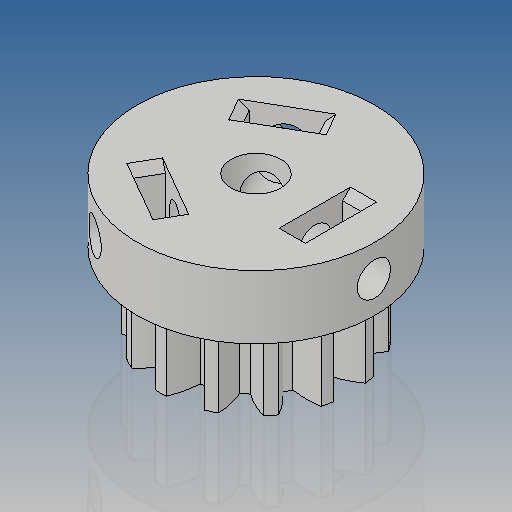
# Autodesk Inventor part: polea
Saved by Autodesk Inventor 2017 (Build 210142000, 142)
## iProperties
Part Number: polea
Material: Genérico
Document SubType Name: Modeling
Designer: Leo
Density: 1 g/cm^3
Appearance: Valor por defecto
Author: Leo
Autodesk Inventor part; units mm, degrees
ref_plane "YZ Plane" through (0, 0, 0) normal (1, 0, 0) x (0, 1, 0)
ref_plane "XZ Plane" through (0, 0, 0) normal (0, 1, 0) x (-1, 0, 0)
ref_plane "XY Plane" through (0, 0, 0) normal (0, 0, 1) x (1, 0, 0)
sketch "Boceto1" plane through (0, 0, 0) normal (0, 1, 0) x (-1, 0, 0)
  circle A0 centre (0, 0) radius 3.15
  circle A1 centre (0, 0) radius 15
  line L0 (-7.425, 3.5) -> (-10.725, 3.5)
  line L1 (-10.725, 3.5) -> (-10.725, -3.5)
  line L2 (-10.725, -3.5) -> (-7.425, -3.5)
  line L3 (-7.425, -3.5) -> (-7.425, 3.5)
  circle A2 centre (0, 0) radius 9.7265 construction
  line L4 (6.7436, -4.6802) -> (0.6814, -8.1802)
  line L5 (8.3936, -7.5381) -> (6.7436, -4.6802)
  line L6 (2.3314, -11.0381) -> (8.3936, -7.5381)
  line L7 (0.6814, -8.1802) -> (2.3314, -11.0381)
  line L8 (0.6814, 8.1802) -> (6.7436, 4.6802)
  line L9 (2.3314, 11.0381) -> (0.6814, 8.1802)
  line L10 (8.3936, 7.5381) -> (2.3314, 11.0381)
  line L11 (6.7436, 4.6802) -> (8.3936, 7.5381)
  point P0 (-7.425, 0)
  point P1 (-9.075, 3.5)
  point P2 (3.7125, -6.4302)
  point P3 (1.5064, -9.6092)
  point P4 (3.7125, 6.4302)
  point P5 (7.5686, 6.1092)
  dimension "d0" = 6.3
  dimension "tuerca" = 7
  dimension "d2" = 11.85
  dimension "d3" = 6.5765
  dimension "d4" = 3.3
  dimension "d18" = 360
  dimension "d26" = 30
  dimension "d27" = 4.275
  dimension "d28" = 4.275
  constraints: 24 end point, 2 centre point, 2 coincident, 2 midpoint, 2 parallel, 1 horizontal, 1 horizontal alignment, 1 perpendicular, 34 other
  measures "d0" diameter of A0
  measures "tuerca" distance of L0.end L1.end
  measures "d2" radial gap between concentric circles of A1 A0
  measures "d4" distance of L0.start L0.end
  measures "d26" diameter of A1
  measures "d27" distance edge to line of A0 L3
  measures "d28" distance edge to line of A1 L1
extrude "Extrusión1" add sketch "Boceto1" along normal blind 8
sketch "Boceto2" plane through (7.425, 0, -3.5) normal (1, 0, 0) x (0, 0, -1)
  line L0 (0, 0) -> (-7, 0) projected
  line L1 (0, 0) -> (0, 8) construction
  line L2 (-7, 8) -> (0, 8) construction
  line L3 (-7, 0) -> (-7, 8) construction
  line L4 (-7, 0) -> (0, 8) construction
  circle A0 centre (-3.5, 4) radius 2.1
  line L5 (0, 1.7483) -> (-3.0282, 0)
  line L6 (-3.9718, 0) -> (-7, 1.7483)
  line L7 (-7, 1.7483) -> (-7, 0)
  line L8 (0, 1.7483) -> (0, 0)
  point P0 (-3.5, 0)
  dimension "d7" = 4.2
  dimension "d8" = 120
  dimension "d9" = 3.7
  constraints: 10 end point, 4 point on line, 1 centre point, 1 collinear, 1 equal length, 1 horizontal alignment, 1 midpoint
  measures "d7" diameter of A0
  measures "d8" angle of L5 L6
  measures "d9" distance from line of A0.centre L5
extrude "Extrusión2" cut sketch "Boceto2" along normal mid plane 16 contours A0
extrude "Extrusión3" add sketch "Boceto2" along normal up to next contours L0 L5 L8 | L0 L7 L6
sketch "Boceto3" plane through (0, 0, 0) normal (0, -1, 0) x (1, 0, 0)
  circle A0 centre (0, 0) radius 3.15 projected
  circle A1 centre (0, 0) radius 17.939
  constraints: 1 centre point
extrude "Extrusión4" add sketch "Boceto3" along normal blind 10
spur gear teeth "iFeature1:3" teeth 14 pitch diameter 21 tip diameter 24 root diameter 17.25 face width 10 trims to tip circle yes start plane through (0, 0, 0) normal (0, 1, 0) x (-1, 0, 0)
pattern_circular "Patrón circular1" count 3 over 360 about axis through (0, -10, 0) along (0, 1, 0) of "Extrusión2", "Extrusión3"
chamfer "Chaflán1" distance 1 angle 45 6 edges at (-1.5064, 8, 9.6092) (-7.5686, 8, 6.1092) (-7.5686, 8, -6.1092) (-1.5064, 8, -9.6092) (9.075, 8, 3.5) (9.075, 8, -3.5)
equation "\"d28\" = d27"
